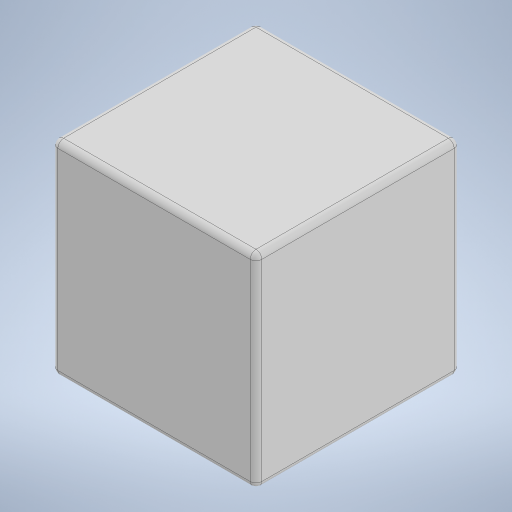
# Autodesk Inventor part: Item
Saved by Autodesk Inventor 2023 (Build 270158000, 158)
## iProperties
Created: 2024-01-19
Part Number: Item
Material: Všeobecné
Document SubType Name: Modeling
Designer: zak
Density: 1 g/cm^3
Appearance: Výchozí
Author: zak
Autodesk Inventor part; units mm, degrees
ref_plane "YZ Plane" through (0, 0, 0) normal (1, 0, 0) x (0, 1, 0)
ref_plane "XZ Plane" through (0, 0, 0) normal (0, 1, 0) x (-1, 0, 0)
ref_plane "XY Plane" through (0, 0, 0) normal (0, 0, 1) x (1, 0, 0)
sketch "Náčrt1" plane through (0, 0, 0) normal (0, 0, 1) x (1, 0, 0)
  line L0 (-24.5, 0) -> (24.5, 0) projected
  line L1 (0, -24.5) -> (0, 24.5) projected
  line L2 (-17.5, 17.5) -> (17.5, 17.5)
  line L3 (17.5, 17.5) -> (17.5, -17.5)
  line L4 (17.5, -17.5) -> (-17.5, -17.5)
  line L5 (-17.5, -17.5) -> (-17.5, 17.5)
  point P0 (0, 0)
  dimension "d0" = 35
  dimension "d1" = 35
  constraints: 8 end point, 2 parallel, 1 horizontal, 1 perpendicular, 2 other
  measures "d0" distance of L3.end L4.end
  measures "d1" distance of L2.end L3.end
extrude "Vysunutí1" add sketch "Náčrt1" along normal blind 35
fillet "Zaoblení1" radius 1 12 edges at (17.5, 17.5, 17.5) (0, 17.5, 35) (17.5, 0, 35) (-17.5, 0, 35) (-17.5, 17.5, 17.5) (-17.5, 0, 0) (0, -17.5, 0) (0, -17.5, 35) (-17.5, -17.5, 17.5) (17.5, 0, 0) (17.5, -17.5, 17.5) (0, 17.5, 0)
equation "\"d1\" = d0"
equation "\"d2\" = d1"
